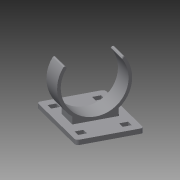
# Autodesk Inventor part: Clip
Saved by Autodesk Inventor 2015 (Build 190159000, 159)
## iProperties
Created: 2018-12-12
Part Number: Clip
Material: Generic
Document SubType Name: Modeling
Designer: 579494
Density: 1 g/cm^3
Appearance: Default
Author: 579494
Autodesk Inventor part; units mm, degrees
ref_plane "YZ Plane" through (0, 0, 0) normal (1, 0, 0) x (0, 1, 0)
ref_plane "XZ Plane" through (0, 0, 0) normal (0, 1, 0) x (-1, 0, 0)
ref_plane "XY Plane" through (0, 0, 0) normal (0, 0, 1) x (1, 0, 0)
sketch "Sketch1" plane through (0, 0, 0) normal (0, 0, 1) x (1, 0, 0)
  arc A0 (19, 0) -> (-5.2482, -18.2608) centre (0, 0) ccw
  line L0 (-5.2482, -18.2608) -> (-5.2482, -20.2608)
  line L1 (19, 0) -> (21, 0)
  arc A1 (21, 0) -> (-5.2482, -20.2608) centre (0.0001, 0.0728) ccw
  line L2 (-12.8316, 16.6965) -> (2.2089, 28.3061)
  line L3 (2.2089, 28.3061) -> (-12.8316, 16.6965)
  line L4 (-12.8316, 16.6965) -> (-27.8721, 5.0869)
  line L5 (-27.8721, 5.0869) -> (-29.7052, 7.4617)
  line L6 (-29.7052, 7.4617) -> (0.3758, 30.681)
  line L7 (0.3758, 30.681) -> (2.2089, 28.3061)
  point P0 (0, 0)
  dimension "d1" = 19
  dimension "d2" = 2
  dimension "d3" = 2
  dimension "d4" = 21
  dimension "d5" = 19
  dimension "d6" = 19
  dimension "d7" = 3
  constraints: 16 end point, 5 point on circle, 2 centre point, 2 perpendicular, 1 collinear, 1 horizontal, 1 point on line, 1 vertical
  measures "d1" radius of A0
  measures "d2" distance of L0.start L0.end
  measures "d3" distance of L1.start L1.end
  measures "d4" radius of A1
  measures "d5" distance of L2.start L2.end
  measures "d6" distance of L2.start L4.end
  measures "d7" distance of L4.end L5.end
extrude "Extrusion1" add sketch "Sketch1" along normal blind 15
sketch "Sketch2" plane through (0, 0, 0) normal (0, 0, -1) x (-1, 0, 0)
  line L0 (29.7052, 7.4617) -> (-0.3758, 30.681)
  line L1 (-0.3758, 30.681) -> (29.7052, 7.4617) projected
  line L2 (-0.3758, 30.681) -> (-2.2089, 28.3061)
  line L3 (-2.2089, 28.3061) -> (27.8721, 5.0869)
  line L4 (27.8721, 5.0869) -> (29.7052, 7.4617)
  point P0 (0, 0)
  constraints: 8 end point, 3 perpendicular, 1 collinear
extrude "Extrusion2" add sketch "Sketch2" along normal blind 20
sketch "Sketch3" plane through (0, 0, 15) normal (0, 0, 1) x (1, 0, 0)
  line L0 (0.3758, 30.681) -> (2.2089, 28.3061)
  line L1 (2.2089, 28.3061) -> (0.3758, 30.681) projected
  line L2 (2.2089, 28.3061) -> (-27.8721, 5.0869)
  line L3 (-27.8721, 5.0869) -> (-12.8316, 16.6965) projected
  line L4 (-27.8721, 5.0869) -> (-29.7052, 7.4617)
  line L5 (-29.7052, 7.4617) -> (0.3758, 30.681)
  point P0 (0, 0)
  constraints: 8 end point, 2 collinear, 2 perpendicular
extrude "Extrusion3" add sketch "Sketch3" along normal blind 20
sketch "Sketch6" plane through (0, 0, 0) normal (0, 0, -1) x (-1, 0, 0)
  line L0 (12.8316, 16.6965) -> (23.1224, 8.7531)
  line L1 (-2.2089, 28.3061) -> (27.8721, 5.0869) projected
  line L2 (23.1224, 8.7531) -> (20.3682, 5.1848)
  arc A0 (5.2482, -20.2608) -> (12.8316, 16.6965) centre (-0.0001, 0.0728) ccw projected
  line L3 (12.8316, 16.6965) -> (2.5407, 24.6399)
  line L4 (2.5407, 24.6399) -> (-0.2136, 21.0717)
  arc A1 (12.8316, 16.6965) -> (-21, 0) centre (-0.0001, 0.0728) ccw projected
  arc A2 (20.3682, 5.1848) -> (12.8316, 16.6965) centre (-0.0001, 0.0728) ccw
  arc A3 (12.8316, 16.6965) -> (-0.2136, 21.0717) centre (-0.0001, 0.0728) ccw
  point P0 (0, 0)
  dimension "d22" = 13
  dimension "d23" = 13
  constraints: 8 end point, 6 point on circle, 2 centre point, 2 perpendicular, 2 point on line, 1 concentric
  measures "d22" distance of L0.start L0.end
  measures "d23" distance of L0.start L3.end
extrude "Extrusion6" add sketch "Sketch6" against normal blind 15
sketch "Sketch7" plane through (-27.8721, 5.0869, -20) normal (0.6110339, -0.7916044, 0) x (0.7916044, 0.6110339, 0)
  line L0 (38, 0) -> (38, 55) projected
  line L1 (4.4154, 49) -> (9.4154, 49)
  line L2 (9.4154, 49) -> (9.4154, 44)
  line L3 (9.4154, 44) -> (4.4154, 44)
  line L4 (4.4154, 44) -> (4.4154, 49)
  line L5 (34.4154, 49) -> (29.4154, 49)
  line L6 (29.4154, 49) -> (29.4154, 44)
  line L7 (29.4154, 44) -> (34.4154, 44)
  line L8 (34.4154, 44) -> (34.4154, 49)
  line L9 (38, 55) -> (38, 27.5)
  line L10 (38, 0) -> (38, 55) projected
  line L11 (38, 27.5) -> (0, 27.5)
  line L12 (0, 0) -> (0, 55) projected
  line L13 (38, 27.5) -> (0, 27.5)
  line L14 (4.4154, 6) -> (9.4154, 6)
  line L15 (9.4154, 6) -> (9.4154, 11)
  line L16 (9.4154, 11) -> (4.4154, 11)
  line L17 (4.4154, 11) -> (4.4154, 6)
  line L18 (34.4154, 6) -> (29.4154, 6)
  line L19 (29.4154, 6) -> (29.4154, 11)
  line L20 (29.4154, 11) -> (34.4154, 11)
  line L21 (34.4154, 11) -> (34.4154, 6)
  point P0 (18.9554, 20)
  dimension "d27" = 5
  dimension "d28" = 5
  dimension "d29" = 5
  dimension "d30" = 20
  dimension "d31" = 27.5
  dimension "d32" = 33
  constraints: 38 end point, 8 symmetric about line, 5 equal length, 2 horizontal, 2 midpoint, 2 perpendicular, 2 point on line
  measures "d27" distance of L2.end L3.end
  measures "d28" distance of L7.end L6.end
  measures "d29" distance of L5.end L6.end
  measures "d30" distance between parallel lines of L2 L6
  measures "d31" distance of L0.end L9.end
  measures "d32" distance between parallel lines of L20 L7
extrude "Extrusion7" cut sketch "Sketch7" against normal blind 15
fillet "Fillet1" radius 2 4 edges at (1.2923, 29.4935, 35) (-28.7886, 6.2743, 35) (1.2923, 29.4935, -20) (-28.7886, 6.2743, -20)
fillet "Fillet2" radius 1 4 edges at (21, 0, 7.5) (19, 0, 7.5) (-5.2482, -20.2608, 7.5) (-5.2482, -19.2608, 15)
body "Solid1"
